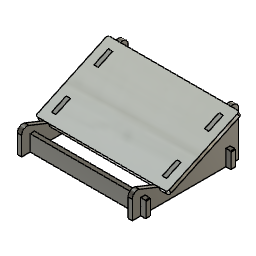
simalokavonandi v12 (Autodesk Fusion 360 design; units mm, degrees)
Autodesk Fusion 360 part; units mm, degrees
note: some values were not read from the file. Set by a fixed rule: which sketch regions a step uses.
sketch "Sketch1" plane through (0, 0, 0) normal (1, 0, 0) x (0, 1, 0) in component "hliðar"
  line L0 (0, 0) -> (0, 25)
  line L1 (100, 50) -> (100, 0)
  line L2 (100, 0) -> (0, 0)
  line L3 (100, 50) -> (24.9423, 15)
  line L4 (24.9423, 15) -> (0, 25)
  dimension "d1" = 50
  dimension "d4" = 25
  dimension "d5" = 100
  dimension "d6" = 15
  dimension "d7" = 65
  constraint coincident L0.start L2.end
  constraint vertical L0
  constraint parallel L0 L1
  constraint perpendicular L0 L2
  measures "d1" distance of L1.start L1.end
  measures "d4" distance of L0.start L0.end
  measures "d5" distance of L1.end L0.start
  measures "d6" distance of L2 L3.end
  measures "d7" angle of L1 L3
extrude "Extrude1" add sketch "Sketch1" along normal blind 4 makes body 1 in component "hliðar"
fillet "Fillet1" radius 5 1 edges at (2, 0, 25) on bodies 1 in component "hliðar"
fillet "Fillet2" radius 5 1 edges at (2, 100, 50) on bodies 1 in component "hliðar"
sketch "Sketch1 (2)" plane through (0, -1.2905, 2.7675) normal (0, -0.422618, 0.906308) x (1, 0, 0) in component "top"
  line L0 (-100, 28.9446) -> (-100, 103.9133)
  line L1 (-100, 103.9133) -> (-104, 103.9133)
  line L2 (-104, 103.9133) -> (-104, 28.9446)
  line L3 (4, 28.9446) -> (4, 103.9133)
  line L4 (4, 103.9133) -> (0, 103.9133)
  line L5 (0, 103.9133) -> (0, 28.9446)
  line L6 (12, 28.9446) -> (-112, 28.9446)
  line L7 (-112, 28.9446) -> (-112, 103.9133)
  line L8 (-112, 103.9133) -> (12, 103.9133)
  line L9 (12, 103.9133) -> (12, 28.9446)
  line L10 (-50, 103.9133) -> (-50, 28.9446) construction
  line L11 (-112, 66.429) -> (12, 66.429) construction
  line L12 (0, 95.8339) -> (4, 95.8339)
  line L13 (4, 95.8339) -> (4, 80.8339)
  line L14 (4, 80.8339) -> (0, 80.8339)
  line L15 (0, 80.8339) -> (0, 95.8339)
  line L16 (-100, 80.8339) -> (-100, 95.8339)
  line L17 (-100, 95.8339) -> (-104, 95.8339)
  line L18 (-104, 80.8339) -> (-100, 80.8339)
  line L19 (-104, 95.8339) -> (-104, 80.8339)
  line L20 (-104, 37.024) -> (-104, 52.024)
  line L21 (-104, 52.024) -> (-100, 52.024)
  line L22 (-100, 52.024) -> (-100, 37.024)
  line L23 (-100, 37.024) -> (-104, 37.024)
  line L24 (4, 37.024) -> (4, 52.024)
  line L25 (4, 52.024) -> (0, 52.024)
  line L26 (0, 52.024) -> (0, 37.024)
  line L27 (0, 37.024) -> (4, 37.024)
  line L28 (0, 28.9446) -> (0, 15.6209)
  line L29 (0, 15.6209) -> (4, 15.6209)
  line L30 (4, 15.6209) -> (4, 28.9446)
  line L31 (-104, 28.9446) -> (-100, 28.9446)
  line L32 (0, 28.9446) -> (4, 28.9446)
  line L33 (4, 28.9446) -> (0, 28.9446)
  line L34 (0, 0) -> (0, 90.6308)
  line L35 (0, 90.6308) -> (4, 90.6308)
  line L36 (4, 90.6308) -> (4, 0)
  line L37 (4, 0) -> (0, 0)
  dimension "d35" = 8
  dimension "d36" = 8
  dimension "d37" = 15
  constraint horizontal L6
  constraint vertical L7
  constraint horizontal L8
  constraint vertical L9
  constraint midpoint L8 L10.start
  constraint midpoint L6 L10.end
  constraint midpoint L7 L11.start
  constraint midpoint L9 L11.end
  constraint horizontal L12
  constraint vertical L13
  constraint horizontal L14
  constraint vertical L15
  constraint coincident L3 L13.end
  constraint coincident L5 L12.start
  constraint symmetric L10 L12.start L16.end
  constraint symmetric L10 L12.end L17.end
  constraint symmetric L10 L13.end L18.start
  constraint symmetric L10 L14.end L16.start
  constraint symmetric L11 L12.start L26.end
  constraint symmetric L11 L12.end L24.start
  constraint symmetric L11 L13.end L24.end
  constraint symmetric L11 L14.end L25.end
  constraint symmetric L11 L17.end L20.start
  constraint symmetric L11 L16.start L21.end
  constraint symmetric L11 L18.start L20.end
  constraint symmetric L11 L16.end L22.end
  constraint collinear L6 L32
  constraint collinear L4 L8
  measures "d35" distance of L3 L9
  measures "d36" distance of L2 L7
  measures "d37" distance of L12.end L13.end
extrude "Extrude1'" add sketch "Sketch1 (2)" against normal blind 4 separate body contours L0 L2 L6 L23 L31 | L0 L5 L6 L8 L15 L16 L22 L26 L34 | L3 L5 L6 L27 L32 L33 L34 L36 | L2 L6 L7 L8 L19 L20 | L0 L2 L18 L21 | L3 L6 L8 L9 L13 L24 L36 | L3 L5 L14 L25 L34 L36 | L0 L1 L2 L8 L17 | L3 L4 L5 L8 L12 makes body 2 in component "top"
combine "Combine1" operation cut target body 1 tool bodies 2 keep tools in component "hliðar"
fillet "Fillet1'" radius 2 1 edges at (12, 25.7875, 13.1874) on bodies 2 in component "top"
fillet "Fillet2'" radius 2 1 edges at (12, 93.7321, 44.8705) on bodies 2 in component "top"
fillet "Fillet3" radius 2 1 edges at (-112, 25.7875, 13.1874) on bodies 2 in component "top"
fillet "Fillet4" radius 2 1 edges at (-112, 93.7321, 44.8705) on bodies 2 in component "top"
ref_plane "WorkPlane1" through (2, 90, 25) normal (0, 1, 0) x (0, 0, 1) in component "stuðningur bak"
sketch "Sketch1 (3)" plane through (2, 90, 21.0758) normal (0, 1, 0) x (1, 0, 0) in component "stuðningur bak"
  line L0 (-106, -19.8476) -> (-102, -19.8476)
  line L1 (-102, -19.8476) -> (-102, 21.0758)
  line L2 (-102, 21.0758) -> (-106, 21.0758)
  line L3 (-106, 21.0758) -> (-106, -19.8476)
  line L4 (-2, -19.8476) -> (2, -19.8476)
  line L5 (2, -19.8476) -> (2, 21.0758)
  line L6 (2, 21.0758) -> (-2, 21.0758)
  line L7 (-2, 21.0758) -> (-2, -19.8476)
  line L8 (7, 21.0758) -> (-111, 21.0758)
  line L9 (-111, 21.0758) -> (-111, 6.0758)
  line L10 (-111, 6.0758) -> (7, 6.0758)
  line L11 (7, 6.0758) -> (7, 21.0758)
  line L12 (10, -21.1369) -> (10, 8.8558)
  line L13 (-114, 8.8558) -> (-114, -21.1369)
  line L14 (7, 13.5758) -> (-111, 13.5758)
  dimension "d49" = 15
  dimension "d58" = 5
  dimension "d59" = 5
  constraint horizontal L8
  constraint vertical L9
  constraint horizontal L10
  constraint vertical L11
  constraint collinear L6 L8
  constraint midpoint L11 L14.start
  constraint midpoint L9 L14.end
  measures "d49" distance of L8 L10
  measures "d58" distance of L3 L9
  measures "d59" distance of L5 L11
extrude "Extrude1''" add sketch "Sketch1 (3)" along normal mid plane 4 separate body contours L3 L9 L10 L14 | L1 L7 L10 L14 | L3 L8 L9 L14 | L1 L2 L3 L8 L14 | L1 L7 L8 L14 | L5 L6 L7 L8 L14 | L5 L10 L11 L14 | L5 L8 L11 L14 makes body 3 in component "stuðningur bak"
ref_plane "WorkPlane2" through (2, 50, 25) normal (0, 1, 0) x (0, 0, 1) in component "stuðningur bak"
fillet "Fillet3'" radius 0.5 4 edges at (9, 90, 15) (9, 90, 0) (-109, 90, 15) (-109, 90, 0) on bodies 3 in component "stuðningur bak"
mirror "Mirror1" [suppressed] in component "stuðningur bak"
combine "Combine3" operation cut target body 1 tool bodies 3 body 3 seen with x (1, 0, 0) y (0, 1, 0) z (0, 0, 1) at (0, -80, 0) keep tools in component "hliðar"
combine "Combine4" operation cut target body 1 tool bodies 3 keep tools in component "hliðar"
ref_plane "WorkPlane1" through (4, 50, 23.9212) normal (1, 0, 0) x (0, 0, -1) in component "Laser Path - hliðar - Body1"
sketch "Path Offsets" plane through (4, 0, 0) normal (1, 0, 0) x (0, 0, -1) in component "Laser Path - hliðar - Body1"
  line L0 (-7.5, 92) -> (0, 92)
  line L1 (0, 92) -> (0, 100)
  line L2 (0, 100) -> (-42.1516, 100)
  arc A0 (-42.1516, 100) -> (-46.6831, 92.8869) centre (-42.1516, 95) ccw
  line L3 (-46.6831, 92.8869) -> (-43.0579, 94.5774)
  line L4 (-43.0579, 94.5774) -> (-39.6434, 87.255)
  line L5 (-39.6434, 87.255) -> (-43.2686, 85.5645)
  line L6 (-43.2686, 85.5645) -> (-36.9293, 71.9699)
  line L7 (-36.9293, 71.9699) -> (-33.3041, 73.6603)
  line L8 (-33.3041, 73.6603) -> (-21.1285, 47.5498)
  line L9 (-21.1285, 47.5498) -> (-24.7538, 45.8593)
  line L10 (-24.7538, 45.8593) -> (-18.4145, 32.2647)
  line L11 (-18.4145, 32.2647) -> (-14.7893, 33.9552)
  line L12 (-14.7893, 33.9552) -> (-11.3748, 26.6327)
  line L13 (-11.3748, 26.6327) -> (-15, 24.9423)
  line L14 (-15, 24.9423) -> (-22.2494, 6.8607)
  arc A1 (-22.2494, 6.8607) -> (-17.6085, 0) centre (-17.6085, 5) ccw
  line L15 (-17.6085, 0) -> (0, 0)
  line L16 (0, 0) -> (0, 8)
  line L17 (0, 8) -> (-7.5, 8)
  line L18 (-7.5, 8) -> (-7.5, 12)
  line L19 (-7.5, 12) -> (0, 12)
  line L20 (0, 12) -> (0, 88)
  line L21 (0, 88) -> (-7.5, 88)
  line L22 (-7.5, 88) -> (-7.5, 92)
  line L23 (0.1035, 91.8965) -> (0.1035, 100.1035)
  line L24 (0.1035, 100.1035) -> (-42.1516, 100.1035)
  arc A2 (-42.1516, 100.1035) -> (-46.7322, 92.7498) centre (-42.1516, 95) ccw
  line L25 (-46.7322, 92.7498) -> (-43.1079, 94.4398)
  line L26 (-43.1079, 94.4398) -> (-39.7809, 87.305)
  line L27 (-39.7809, 87.305) -> (-43.4062, 85.6145)
  line L28 (-43.4062, 85.6145) -> (-36.9794, 71.8323)
  line L29 (-36.9794, 71.8323) -> (-33.3542, 73.5228)
  line L30 (-33.3542, 73.5228) -> (-21.2661, 47.5998)
  line L31 (-21.2661, 47.5998) -> (-24.8913, 45.9094)
  line L32 (-24.8913, 45.9094) -> (-18.4646, 32.1271)
  line L33 (-18.4646, 32.1271) -> (-14.8393, 33.8176)
  line L34 (-14.8393, 33.8176) -> (-11.5123, 26.6828)
  line L35 (-11.5123, 26.6828) -> (-15.0808, 25.0188)
  line L36 (-15.0808, 25.0188) -> (-22.3455, 6.8992)
  arc A3 (-22.3455, 6.8992) -> (-17.6085, -0.1035) centre (-17.6085, 5) ccw
  line L37 (-17.6085, -0.1035) -> (0.1035, -0.1035)
  line L38 (0.1035, -0.1035) -> (0.1035, 8.1035)
  line L39 (0.1035, 8.1035) -> (-7.3965, 8.1035)
  line L40 (-7.3965, 8.1035) -> (-7.3965, 11.8965)
  line L41 (-7.3965, 11.8965) -> (0.1035, 11.8965)
  line L42 (0.1035, 11.8965) -> (0.1035, 88.1035)
  line L43 (0.1035, 88.1035) -> (-7.3965, 88.1035)
  line L44 (-7.3965, 88.1035) -> (-7.3965, 91.8965)
  line L45 (-7.3965, 91.8965) -> (0.1035, 91.8965)
  dimension "d84" = 0.1035
sketch "Perimeter" plane through (4, 50, 23.9212) normal (1, 0, 0) x (0, 0, -1) in component "Laser Path - hliðar - Body1"
  line L0 (8.8404, -24.9812) -> (1.5757, -43.1008)
  arc A0 (1.5757, -43.1008) -> (6.3127, -50.1035) centre (6.3127, -45) ccw
  line L1 (6.3127, -50.1035) -> (24.0247, -50.1035)
  line L2 (24.0247, -50.1035) -> (24.0247, -41.8965)
  line L3 (24.0247, -41.8965) -> (16.5247, -41.8965)
  line L4 (16.5247, -41.8965) -> (16.5247, -38.1035)
  line L5 (16.5247, -38.1035) -> (24.0247, -38.1035)
  line L6 (24.0247, -38.1035) -> (24.0247, 38.1035)
  line L7 (24.0247, 38.1035) -> (16.5247, 38.1035)
  line L8 (16.5247, 38.1035) -> (16.5247, 41.8965)
  line L9 (16.5247, 41.8965) -> (24.0247, 41.8965)
  line L10 (24.0247, 41.8965) -> (24.0247, 50.1035)
  line L11 (24.0247, 50.1035) -> (-18.2304, 50.1035)
  arc A1 (-18.2304, 50.1035) -> (-22.811, 42.7498) centre (-18.2304, 45) ccw
  line L12 (-22.811, 42.7498) -> (-19.1867, 44.4398)
  line L13 (-19.1867, 44.4398) -> (-15.8597, 37.305)
  line L14 (-15.8597, 37.305) -> (-19.485, 35.6145)
  line L15 (-19.485, 35.6145) -> (-13.0582, 21.8323)
  line L16 (-13.0582, 21.8323) -> (-9.433, 23.5228)
  line L17 (-9.433, 23.5228) -> (2.6551, -2.4002)
  line L18 (2.6551, -2.4002) -> (-0.9701, -4.0906)
  line L19 (-0.9701, -4.0906) -> (5.4566, -17.8729)
  line L20 (5.4566, -17.8729) -> (9.0819, -16.1824)
  line L21 (9.0819, -16.1824) -> (12.4089, -23.3172)
  line L22 (12.4089, -23.3172) -> (8.8404, -24.9812)
sketch "Cutouts" plane through (4, 50, 23.9212) normal (1, 0, 0) x (0, 0, -1) in component "Laser Path - hliðar - Body1"
component "3d model" placed x (1, 0, 0) y (0, 1, 0) z (0, 0, 1) at (0, 0, 0)
component "Laser Path - hliðar - Body1" placed x (1, 0, 0) y (0, 1, 0) z (0, 0, 1) at (0, 0, 0)
component "hliðar" placed x (1, 0, 0) y (0, 1, 0) z (0, 0, 1) at (-104, 0, 0) in component "3d model"
component "hliðar" placed x (1, 0, 0) y (0, 1, 0) z (0, 0, 1) at (0, 0, 0) in component "3d model"
component "top" placed x (1, 0, 0) y (0, 1, 0) z (0, 0, 1) at (0, 0, 0) in component "3d model"
component "stuðningur bak" placed x (1, 0, 0) y (0, 1, 0) z (0, 0, 1) at (0, 0, 0) in component "3d model"
component "stuðningur bak" placed x (1, 0, 0) y (0, 1, 0) z (0, 0, 1) at (0, -80, 0) in component "3d model"
equation "d1 = hæðhlið"
equation "d4 = hæðhlið / 2"
equation "d5 = lengdhlið"
equation "d6 = stærðfinger"
equation "d7 = storthornhlið"
equation "hæðhlið = 50 mm"
equation "lengdhlið = 100 mm"
equation "storthornhlið = 65 deg"
equation "þykkthliðar = 4 mm"
equation "d14 = þykkthliðar"
equation "d25 = lengdplötu"
equation "lengdplötu = 100 mm"
equation "stærðfinger = 15 mm"
equation "d35 = þykkthliðar * 2"
equation "d36 = þykkthliðar * 2"
equation "d37 = stærðfinger"
equation "d38 = -þykkthliðar"
equation "d49 = stærðfinger"
equation "d50 = þykkthliðar / 2"
equation "d58 = stuðningur_utur"
equation "d59 = stuðningur_utur"
equation "millistuðnings = -80 mm"
equation "stuðningur_utur = 5 mm"
equation "offset = 0.00 mm"
